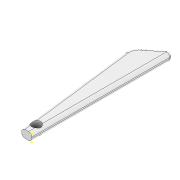
# Autodesk Inventor part: cock clamp
Saved by Autodesk Inventor 2021 (Build 250183000, 183)
## iProperties
Created: 2021-06-21
Part Number: cock clamp
Material: PC/ABS Plastic
Document SubType Name: Modeling
Designer: user
Density: 0.357273 g/cm^3
Appearance: Smooth - White
Author: user
Autodesk Inventor part; units mm, degrees
ref_plane "YZ Plane" through (0, 0, 0) normal (1, 0, 0) x (0, 1, 0)
ref_plane "XZ Plane" through (0, 0, 0) normal (0, 1, 0) x (-1, 0, 0)
ref_plane "XY Plane" through (0, 0, 0) normal (0, 0, 1) x (1, 0, 0)
sketch "Sketch1" plane through (0, 0, 0) normal (0, 1, 0) x (-1, 0, 0)
  line L0 (0, 0) -> (12.7, 0)
  line L1 (0, -129.6628) -> (0, 0)
  line L2 (0, -129.6628) -> (0, -142.3628)
  line L3 (0, -142.3628) -> (16.3017, -129.6628)
  line L4 (0, 0) -> (6.35, 0)
  line L5 (16.3017, -129.6628) -> (25.047, -123.1227)
  line L6 (6.35, 0) -> (18.1234, 0)
  line L7 (9.9069, 0) -> (25.047, -123.1227)
  circle A0 centre (4.9306, -5.8204) radius 4.445
  dimension "d10" = 8.89
  constraints: 16 end point, 3 coincident, 2 point on line, 1 centre point, 1 collinear, 1 horizontal, 1 midpoint
  measures "d10" diameter of A0
sketch "Sketch2" plane through (0, 0, 0) normal (0, 1, 0) x (-1, 0, 0)
  point P0 (0, 0)
extrude "Extrusion1" add sketch "Sketch1" along normal blind 7.62 contours L0 L7 L5 L3 L2 L1 | A0
fillet "Fillet1" radius 25.4 1 edges at (-16.3017, 3.81, -129.6628)
sketch "Sketch3" plane through (0, 7.62, 0) normal (0, 1, 0) x (1, 0, 0)
  point P0 (0, 0)
sketch "Sketch4" plane through (0, 7.62, 0) normal (0, 1, 0) x (1, 0, 0)
  point P0 (0, 0)
sketch "Sketch5" plane through (0, 7.62, 0) normal (0, 1, 0) x (1, 0, 0)
  circle A0 centre (-5.6716, 10.0387) radius 4.5085
  point P0 (0, 0)
  dimension "d11" = 9.017
  constraints: 1 centre point
  measures "d11" diameter of A0
extrude "Extrusion2" cut sketch "Sketch5" against normal through all
fillet "Fillet2" radius 12.7 1 edges at (-25.047, 3.81, -123.1227)
fillet "Fillet3" radius 3.175 1 edges at (0, 3.81, -142.3628)
fillet "Fillet4" radius 3.175 12 edges at (-1.7812, 0, -138.7172) (-10.6152, 0, -134.0929) (-17.8257, 0, -128.5231) (-23.2248, 0, -122.3455) (-17.0275, 0, -57.9065) (0, 0, -67.9322) (-1.7812, 7.62, -138.7172) (-10.6152, 7.62, -134.0929) (-17.8257, 7.62, -128.5231) (-23.2248, 7.62, -122.3455) (-17.0275, 7.62, -57.9065) (0, 7.62, -67.9322)
body "Solid1"
